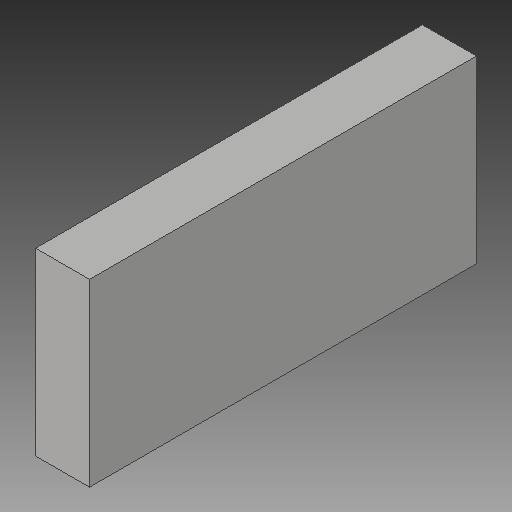
# Autodesk Inventor part: MotorHolderLongAxisTop
Saved by Autodesk Inventor 2018 (Build 220112000, 112)
## iProperties
Created: 2017-10-24
Part Number: MotorHolderLongAxisTop
Material: Generic
Document SubType Name: Modeling
Designer: m228540
Density: 1 g/cm^3
Appearance: Default
Mass: 39.5835 g
Surface Area: 110.35 cm^2
Volume: 39.5835 cm^3
Author: m228540
Autodesk Inventor part; units mm, degrees
ref_plane "YZ Plane" through (0, 0, 0) normal (1, 0, 0) x (0, 1, 0)
ref_plane "XZ Plane" through (0, 0, 0) normal (0, 1, 0) x (-1, 0, 0)
ref_plane "XY Plane" through (0, 0, 0) normal (0, 0, 1) x (1, 0, 0)
sketch "Sketch1" plane through (0, 0, 0) normal (1, 0, 0) x (0, 1, 0)
  line L0 (20, 43) -> (-20, 43)
  line L1 (-20, 43) -> (-20, -43)
  line L2 (-20, -43) -> (20, -43)
  line L3 (20, -43) -> (20, 43)
  line L4 (20, 43) -> (-20, -43) construction
  line L5 (-20, 43) -> (20, -43) construction
  point P0 (0, 0)
  dimension "d0" = 40
  dimension "d1" = 86
  constraints: 12 end point, 2 midpoint, 2 parallel, 1 horizontal, 1 perpendicular
  measures "d0" distance of L0.start L0.end
  measures "d1" distance of L2.end L0.start
extrude "Extrusion1" add sketch "Sketch1" along normal blind 12
sketch "Sketch2" plane through (0, -20, -43) normal (0, -1, 0) x (1, 0, 0)
  circle A0 centre (6, 56) radius 3
  circle A1 centre (6, 76) radius 3
  line L0 (0, 86) -> (12, 86) projected
  line L1 (6, 86) -> (6, 56) construction
  point P0 (0, 43)
  dimension "d4" = 6
  dimension "d6" = 10
  dimension "d7" = 20
  constraints: 2 centre point, 2 end point, 1 equal radius, 1 midpoint, 1 point on line, 1 vertical
  measures "d4" diameter of A1
  measures "d6" distance from line of L0 A1.centre
  measures "d7" distance of A1.centre L1.end
extrude "Extrusion2" cut sketch "Sketch2" against normal blind 15
sketch "Sketch3" plane through (0, -20, -43) normal (0, 0, -1) x (-1, 0, 0)
  line L0 (0, 40) -> (-12, 40) projected
  line L1 (-6, 40) -> (-6, 0) construction
  line L2 (0, 0) -> (-12, 0) projected
  circle A0 centre (-6, 30) radius 3
  circle A1 centre (-6, 10) radius 3
  point P0 (0, 20)
  dimension "d10" = 6
  dimension "d11" = 10
  dimension "d12" = 20
  constraints: 2 centre point, 2 end point, 2 midpoint, 2 point on line, 1 equal radius
  measures "d10" diameter of A1
  measures "d11" distance from line of L2 A1.centre
  measures "d12" distance of A0.centre A1.centre
extrude "Extrusion3" cut sketch "Sketch3" against normal blind 15
thread "Thread1" size "M6x1" class "6H" standard "ANSI Metric M Profile" full length
thread "Thread2" size "M6x1" class "6H" standard "ANSI Metric M Profile" full length
thread "Thread3" size "M6x1" class "6H" standard "ANSI Metric M Profile" full length
thread "Thread4" size "M6x1" class "6H" standard "ANSI Metric M Profile" full length
body "Solid1"
